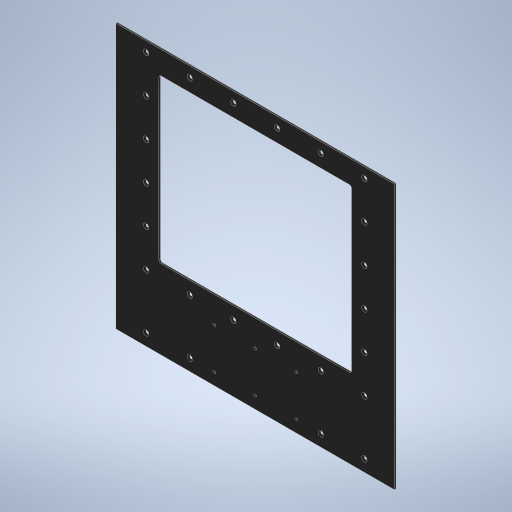
# Autodesk Inventor part: Door Panel R2
Saved by Autodesk Inventor 2024 (Build 280153000, 153)
## iProperties
Created: 2024-09-03
Part Number: Door Panel R2
Material: PET Plastic
Document SubType Name: Modeling
Designer: Ishaan
Density: 1.541 g/cm^3
Appearance: Polycarbonate - Clear
Author: Ishaan
Autodesk Inventor part; units mm, degrees
ref_plane "YZ Plane" through (0, 0, 0) normal (1, 0, 0) x (0, 1, 0)
ref_plane "XZ Plane" through (0, 0, 0) normal (0, 1, 0) x (-1, 0, 0)
ref_plane "XY Plane" through (0, 0, 0) normal (0, 0, 1) x (1, 0, 0)
sketch "Sketch1" plane through (0, 0, 0) normal (0, 0, 1) x (1, 0, 0)
  line L0 (255.5, -242.5) -> (-255.5, -242.5)
  line L1 (-255.5, -242.5) -> (-255.5, 242.5)
  line L2 (-255.5, 242.5) -> (255.5, 242.5)
  line L3 (255.5, 242.5) -> (255.5, -242.5)
  line L4 (255.5, -242.5) -> (-255.5, 242.5) construction
  line L5 (-255.5, -242.5) -> (255.5, 242.5) construction
  point P0 (0, 0)
  dimension "d0" = 511
  dimension "d1" = 485
  constraints: 12 end point, 2 midpoint, 2 parallel, 1 horizontal, 1 perpendicular
  measures "d0" distance of L1.end L2.end
  measures "d1" distance of L0.end L1.end
extrude "Extrusion1" add sketch "Sketch1" against normal blind 3
sketch "Sketch4" plane through (0, 0, 0) normal (0, 0, 1) x (1, 0, 0)
  line L0 (188, -109.15) -> (-188, -109.15)
  line L1 (-188, -109.15) -> (-188, 211.85)
  line L2 (-188, 211.85) -> (188, 211.85)
  line L3 (188, 211.85) -> (188, -109.15)
  line L4 (188, -109.15) -> (-188, 211.85) construction
  line L5 (-188, -109.15) -> (188, 211.85) construction
  line L6 (-200, 223.85) -> (200, 223.85) construction
  line L7 (-200, -121.15) -> (200, -121.15) construction
  line L8 (-200, -221.15) -> (200, -221.15) construction
  line L9 (-255.5, -242.5) -> (255.5, -242.5) projected
  line L10 (0, -121.15) -> (0, 223.85) construction
  line L11 (-200, 154.85) -> (-200, -52.15) construction
  line L12 (200, 154.85) -> (200, -52.15) construction
  line L13 (-200, 51.35) -> (200, 51.35) construction
  line L14 (-255.5, -242.5) -> (-255.5, 242.5) construction
  line L15 (176.5, 200.35) -> (-176.5, 200.35)
  line L16 (-176.5, 200.35) -> (-176.5, -97.65)
  line L17 (-176.5, -97.65) -> (176.5, -97.65)
  line L18 (176.5, -97.65) -> (176.5, 200.35)
  point P0 (0, 0)
  point P1 (0, -221.15)
  point P2 (-200, 85.85)
  point P3 (200, 85.85)
  point P4 (-200, 16.85)
  point P5 (200, 16.85)
  point P6 (0, 51.35)
  point P7 (-120, 223.85)
  point P8 (-40, 223.85)
  point P9 (40, 223.85)
  point P10 (120, 223.85)
  point P11 (-120, -121.15)
  point P12 (-40, -121.15)
  point P13 (40, -121.15)
  point P14 (120, -121.15)
  point P15 (-120, -221.15)
  point P16 (-40, -221.15)
  point P17 (40, -221.15)
  point P18 (120, -221.15)
  dimension "d18" = 21.35
  dimension "d19" = 100
  dimension "d21" = 445
  dimension "d29" = 400
  dimension "d30" = 12
  dimension "d31" = 12
  dimension "d41" = 69
  dimension "d47" = 12
  dimension "d55" = 69
  dimension "d58" = 11.5
  dimension "d70" = 80
  dimension "d77" = 80
  dimension "d84" = 80
  constraints: 34 end point, 10 coincident, 9 midpoint, 7 horizontal, 5 vertical alignment, 4 parallel, 4 vertical, 3 perpendicular, 2 horizontal alignment, 1 point on line, 24 other
  measures "d18" distance between parallel lines of L8 L9
  measures "d19" distance between parallel lines of L7 L8
  measures "d21" distance between parallel lines of L8 L6
  measures "d29" distance of L8.start L8.end
  measures "d30" distance between parallel lines of L6 L2
  measures "d31" distance between parallel lines of L0 L7
  measures "d41" distance of point (-200, 154.85) point (-200, 85.85)
  measures "d47" distance between parallel lines of L1 L11
  measures "d55" distance of point (-200, 223.85) point (-200, 154.85)
  measures "d58" distance between parallel lines of L2 L15
  measures "d70" distance of point (-200, 223.85) point (-120, 223.85)
  measures "d77" distance of point (-200, -121.15) point (-120, -121.15)
  measures "d84" distance of point (-200, -221.15) point (-120, -221.15)
hole "Hole1" at (-200, 223.85, 0) direction (0, 0, -1) diameter 5.4 end through all countersink diameter 10.4 countersink angle 90
pattern_sketch "Sketch Driven Pattern1" of "Hole1" from (-200, 223.85, 0) copies at (-200, -121.15, 0) at (-200, -221.15, 0) at (-200, 154.85, 0) at (200, 154.85, 0) at (-200, 85.85, 0) at (200, 85.85, 0) at (-200, 16.85, 0) at (200, 16.85, 0) at (-200, -52.15, 0) at (200, -52.15, 0) at (-120, 223.85, 0) at (-40, 223.85, 0) at (40, 223.85, 0) at (120, 223.85, 0) at (200, 223.85, 0) at (-120, -121.15, 0) at (-40, -121.15, 0) at (40, -121.15, 0) at (120, -121.15, 0) at (200, -121.15, 0) at (-120, -221.15, 0) at (120, -221.15, 0) at (200, -221.15, 0)
extrude "Extrusion4" cut sketch "Sketch4" against normal through all contours L18 L17 L16 L15
fillet "Fillet2" radius 4 4 edges at (-176.5, -97.65, -1.5) (176.5, -97.65, -1.5) (176.5, 200.35, -1.5) (-176.5, 200.35, -1.5)
sketch "Sketch5" plane through (0, 0, 0) normal (0, 0, 1) x (1, 0, 0)
  line L0 (-200, -121.15) -> (200, -121.15) construction
  line L1 (-200, -221.15) -> (200, -221.15) construction
  line L2 (75, -221.15) -> (-75, -221.15) construction
  line L3 (-75, -221.15) -> (-75, -146.15) construction
  line L4 (-75, -146.15) -> (75, -146.15) construction
  line L5 (75, -146.15) -> (75, -221.15) construction
  line L6 (75, -221.15) -> (-75, -146.15) construction
  line L7 (-75, -221.15) -> (75, -146.15) construction
  point P0 (0, 0)
  point P1 (0, -183.65)
  point P2 (0, -221.15)
  point P3 (0, -221.15)
  point P4 (0, -146.15)
  dimension "d89" = 150
  dimension "d90" = 75
  constraints: 12 end point, 5 coincident, 5 midpoint, 2 parallel, 1 horizontal, 1 perpendicular
  measures "d89" distance of L3.end L4.end
  measures "d90" distance of L2.end L3.end
hole "Hole2" at (-75, -146.15, 0) at (0, -146.15, 0) at (75, -146.15, 0) at (75, -221.15, 0) at (0, -221.15, 0) at (-75, -221.15, 0) direction (0, 0, -1) diameter 5.3 end through all
equation "\"d41\" = d55"
equation "\"d47\" = d30"
body "Solid1"
